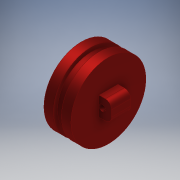
# Autodesk Inventor part: PayloadGermination_SyringePlunger
Saved by Autodesk Inventor 2018 (Build 220112000, 112)
## iProperties
Created: 2018-07-29
Part Number: PayloadGermination_SyringePlunger
Material: Aluminum 6061
Document SubType Name: Modeling
Designer: Bradley
Density: 2.7 g/cm^3
Appearance: Anodized - Red
Author: Bradley
Autodesk Inventor part; units mm, degrees
ref_plane "YZ Plane" through (0, 0, 0) normal (1, 0, 0) x (0, 1, 0)
ref_plane "XZ Plane" through (0, 0, 0) normal (0, 1, 0) x (-1, 0, 0)
ref_plane "XY Plane" through (0, 0, 0) normal (0, 0, 1) x (1, 0, 0)
sketch "Sketch1" plane through (0, 0, 0) normal (0, 1, 0) x (-1, 0, 0)
  line L0 (3.8975, 0) -> (0.3525, 5.9)
  line L1 (0.3525, 5.9) -> (-1.1475, 5.9)
  line L2 (-1.1475, 5.9) -> (-1.1475, 5.25)
  line L3 (-1.1475, 5.25) -> (-2.3975, 5.25)
  line L4 (-2.3975, 5.25) -> (-2.3975, 5.9)
  line L5 (-2.3975, 5.9) -> (-3.8975, 5.9)
  line L6 (-3.8975, 5.9) -> (-3.8975, 0)
  line L7 (-3.8975, 0) -> (3.8975, 0)
  point P0 (0, 0)
  point P1 (0, 0)
  dimension "d0" = 11.8
  dimension "d1" = 1.25
  dimension "d2" = 10.5
  dimension "d3" = 59
  dimension "d4" = 1.5
  constraints: 17 end point, 4 perpendicular, 2 point on line, 1 coincident, 1 collinear, 1 horizontal, 1 midpoint
  measures "d0" diameter of L5 L7
  measures "d1" distance of L2.end L3.end
  measures "d2" diameter of L3 L7
  measures "d3" angle of L7 L0
  measures "d4" distance of L0.end L1.end
revolve "Revolution1" add sketch "Sketch1" angle 360 about axis through (3.8975, 0, 0) along (-1, 0, 0)
sketch "Sketch2" plane through (3.8975, 0, 0) normal (1, 0, 0) x (0, 0, -1)
  line L0 (1.5, -1.5) -> (-1.5, -1.5)
  line L1 (-1.5, -1.5) -> (-1.5, 1.5)
  line L2 (-1.5, 1.5) -> (1.5, 1.5)
  line L3 (1.5, 1.5) -> (1.5, -1.5)
  line L4 (1.5, -1.5) -> (-1.5, 1.5) construction
  line L5 (-1.5, -1.5) -> (1.5, 1.5) construction
  point P0 (0, 0)
  dimension "d6" = 3
  dimension "d7" = 3
  constraints: 12 end point, 2 midpoint, 2 parallel, 1 horizontal, 1 perpendicular
  measures "d6" distance of L1.end L2.end
  measures "d7" distance of L0.end L1.end
extrude "Extrusion1" add sketch "Sketch2" along normal blind 2
sketch "Sketch3" plane through (3.8975, -1.5, -1.5) normal (0, -1, 0) x (1, 0, 0)
  line L0 (0, 0) -> (0, 3) projected
  line L1 (0, 0) -> (2, 0) projected
  line L2 (2, 3) -> (2, 0) projected
  line L3 (0, 3) -> (2, 3) projected
  circle A0 centre (0.5, 1.5) radius 0.5
  line L4 (0, 7.4) -> (0, -4.4) projected
  point P0 (-3.8975, 1.5)
  dimension "d10" = 1
  constraints: 1 centre point, 1 horizontal alignment, 1 tangent
  measures "d10" diameter of A0
extrude "Extrusion2" cut sketch "Sketch3" against normal through all contours A0
fillet "Fillet1" radius 1 2 edges at (5.8975, 0, 1.5) (5.8975, 0, -1.5)
body "Solid1"
